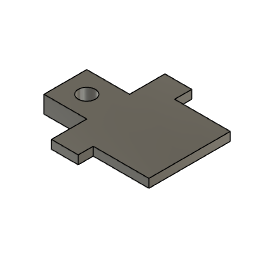
D1Holding (Autodesk Fusion 360 design; units mm, degrees)
Autodesk Fusion 360 part; units mm, degrees
sketch "Sketch1" plane through (0, 0, 0) normal (0, 0, 1) x (1, 0, 0)
  line L0 (0, 0) -> (8.5, 0)
  line L1 (8.5, 0) -> (8.5, 10)
  line L2 (8.5, 10) -> (0, 10)
  line L3 (0, 10) -> (0, 0)
  line L4 (0, 10) -> (10, 10)
  line L5 (10, 10) -> (10, 0)
  line L6 (10, 0) -> (0, 0)
  line L7 (0, 0) -> (0, 10)
  line L8 (0, 10) -> (10, 0)
  line L9 (0, 0) -> (10, 10)
  circle A0 centre (5, 5) radius 2
  dimension "d1" = 8.5
  dimension "d2" = 10
  dimension "d3" = 10
  dimension "d4" = 10
  dimension "d5" = 4
  constraint horizontal L0
  constraint vertical L1
  constraint horizontal L2
  constraint vertical L3
  constraint coincident L0.start L3.end
  constraint horizontal L4
  constraint vertical L5
  constraint horizontal L6
  constraint vertical L7
  constraint midpoint L8 A0.centre
  measures "d1" distance of L0.start L0.end
  measures "d2" distance of L0.start L2.end
  measures "d3" distance of L2.end L4.end
  measures "d4" distance of L2.end L0.start
  measures "d5" diameter of A0
extrude "Extrude1" add sketch "Sketch1" along normal blind 2 contours L0 L1 L6 L8 L9 A0 | L3 L7 L8 L9 A0 | L1 L2 L4 L8 L9 A0 | L1 L8 L9 A0
sketch "Sketch2" plane through (0, 0, 2) normal (0, 0, 1) x (-1, 0, 0)
  circle A0 centre (-5, -5) radius 2
  line L0 (-8.5, 0) -> (-8.5, -10)
  line L1 (-8.5, -10) -> (0, -10)
  line L2 (0, -10) -> (0, 0)
  line L3 (0, 0) -> (-8.5, 0)
  line L4 (-8.5, -10) -> (-10, -10)
  line L5 (-10, -10) -> (-10, 0)
  line L6 (-10, 0) -> (-8.5, 0)
  line L7 (-8.5, 0) -> (-8.5, -10)
  line L8 (-10, -5) -> (-10, -18.25)
  line L9 (-10, -18.25) -> (-10, 8.25)
  line L10 (-10, -18.25) -> (-16.26, -18.25)
  line L11 (-16.26, -18.25) -> (-16.26, 8.25)
  line L12 (-16.26, 8.25) -> (-10, 8.25)
  line L13 (-10, 8.25) -> (-10, -18.25)
  line L14 (-16.26, 8.25) -> (-16.26, 4.75)
  line L15 (-16.26, 4.75) -> (-29.26, 4.75)
  line L16 (-29.26, 4.75) -> (-29.26, -14.25)
  line L17 (-29.26, -14.25) -> (-16.26, -14.25)
  line L18 (-16.26, -14.25) -> (-16.26, 4.75)
  dimension "d8" = 1.5
  dimension "d9" = 13.25
  dimension "d10" = 26.5
  dimension "d11" = 6.26
  dimension "d12" = 26.5
  dimension "d13" = 3.5
  dimension "d14" = 13
  dimension "d15" = 19
  constraint horizontal L4
  constraint vertical L5
  constraint horizontal L6
  constraint vertical L7
  constraint coincident L0.end L1.start
  constraint midpoint L5 L8.start
  constraint parallel L5 L8
  constraint parallel L8 L9
  constraint horizontal L10
  constraint vertical L11
  constraint horizontal L12
  constraint vertical L13
  constraint perpendicular L12 L14
  constraint horizontal L15
  constraint vertical L16
  constraint horizontal L17
  constraint vertical L18
  measures "d8" distance of L0.end L4.end
  measures "d9" distance of L8.start L8.end
  measures "d10" distance of L8.end L9.end
  measures "d11" distance of L8.end L10.end
  measures "d12" distance of L8.end L9.end
  measures "d13" distance of L11.end L14.end
  measures "d14" distance of L14.end L15.end
  measures "d15" distance of L14.end L17.end
extrude "Extrude2" add sketch "Sketch2" along normal blind 2
